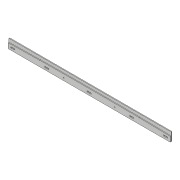
# Autodesk Inventor part: Guia eliptica
Saved by Autodesk Inventor 2019 (Build 230136000, 136)
## iProperties
Created: 2019-11-01
Part Number: Guia eliptica
Material: Generic
Document SubType Name: Modeling
Designer: Charlie
Density: 1 g/cm^3
Appearance: Default
Author: Charlie
Autodesk Inventor part; units mm, degrees
ref_plane "YZ Plane" through (0, 0, 0) normal (1, 0, 0) x (0, 1, 0)
ref_plane "XZ Plane" through (0, 0, 0) normal (0, 1, 0) x (-1, 0, 0)
ref_plane "XY Plane" through (0, 0, 0) normal (0, 0, 1) x (1, 0, 0)
sketch "Sketch1" plane through (0, 0, 0) normal (0, 0, 1) x (1, 0, 0)
  line L0 (-327.5, -120) -> (327.5, -120) construction
  line L1 (327.5, -120) -> (327.5, 120) construction
  line L2 (181.0324, 120) -> (-327.5, 120) construction
  line L3 (-327.5, 120) -> (-327.5, -120) construction
  line L4 (-327.5, -120) -> (327.5, 120) construction
  line L5 (327.5, -120) -> (-327.5, 120) construction
  line L6 (-327.5, 120) -> (-327.5, 122.5) construction
  line L7 (-145.4605, 120) -> (327.5, 120) construction
  line L8 (327.5, 120) -> (327.5, 125.5) construction
  line L9 (327.5, 125.5) -> (-327.5, 125.5) construction
  line L10 (-327.5, 125.5) -> (-327.5, 120) construction
  line L11 (-363.5951, 121.3114) -> (-639.7444, 121.118)
  line L12 (-327.5, 122.5) -> (-344.4955, 122.5)
  ellipse E0 centre (0, 122.5) end of major axis (-327.5, 122.5) minor radius 3 (327.5, 122.5) -> (-327.5, 122.5) ccw
  line L13 (-477.5, 120.5) -> (-292.2253, 123.8544)
  line L14 (-477.5, 120.5) -> (-477.5, 90.5)
  line L15 (-477.5, 90.5) -> (477.5, 90.5)
  line L16 (477.5, 90.5) -> (477.5, 120.5)
  line L17 (477.5, 120.5) -> (292.2253, 123.8544)
  point P0 (0, 0)
  dimension "d1" = 240
  dimension "d2" = 2.5
  dimension "d3" = 5.5
  dimension "d31" = 3
  dimension "d32" = 655
  dimension "d36" = 30
  dimension "d37" = 150
  dimension "d38" = 150
  dimension "d39" = 5
  constraints: 36 end point, 5 parallel, 4 horizontal, 4 perpendicular, 2 horizontal alignment, 2 midpoint, 2 point on line, 1 vertical, 8 other
  measures "d1" distance of L1.end L0.end
  measures "d2" distance of L6.end L2.end
  measures "d3" distance of L8.end L7.end
  measures "d31" distance from line of L6.end L9
  measures "d32" distance of L8.end L9.end
  measures "d36" distance of L13.start L14.end
  measures "d37" distance between parallel lines of L6 L14
  measures "d38" distance between parallel lines of L1 L16
  measures "d39" distance from line of L9 L16.end
extrude "Extrusion1" add sketch "Sketch1" along normal blind 5
sketch "Sketch9" plane through (0, 0, 0) normal (0, 0, -1) x (-1, 0, 0)
  line L0 (477.5, 120.5) -> (292.2253, 123.8544) projected
  ellipse E0 centre (0, 122.5) end of major axis (-327.5, 122.5) minor radius 3 (292.2253, 123.8544) -> (-292.2253, 123.8544) ccw projected
  line L1 (-292.2253, 123.8544) -> (-477.5, 120.5) projected
  line L2 (-477.5, 120.5) -> (-477.5, 90.5) projected
  line L3 (-477.5, 90.5) -> (477.5, 90.5) projected
  line L4 (477.5, 90.5) -> (477.5, 120.5) projected
  line L5 (477.5, 120.5) -> (477.5, 90.5) projected
  line L6 (477.5, 90.5) -> (-477.5, 90.5)
  line L7 (-477.5, 90.5) -> (-477.5, 140.5)
  line L8 (-477.5, 140.5) -> (477.5, 140.5)
  line L9 (477.5, 140.5) -> (477.5, 90.5)
  point P0 (0, 0)
  dimension "d40" = 50
  constraints: 8 end point, 2 parallel, 1 horizontal, 1 perpendicular, 1 other
  measures "d40" distance of L6.end L7.end
extrude "Extrusion7" add sketch "Sketch9" along normal blind 5 separate body
sketch "Sketch10" plane through (0, 0, 5) normal (0, 0, 1) x (1, 0, 0)
  line L0 (-10, 105.5) -> (10, 105.5) construction
  line L1 (-10, 102.5) -> (10, 102.5)
  line L2 (10, 108.5) -> (-10, 108.5)
  arc A0 (-10, 108.5) -> (-10, 102.5) centre (-10, 105.5) ccw
  arc A1 (10, 102.5) -> (10, 108.5) centre (10, 105.5) ccw
  line L3 (240, 105.5) -> (260, 105.5) construction
  line L4 (240, 102.5) -> (260, 102.5)
  line L5 (260, 108.5) -> (240, 108.5)
  arc A2 (240, 108.5) -> (240, 102.5) centre (240, 105.5) ccw
  arc A3 (260, 102.5) -> (260, 108.5) centre (260, 105.5) ccw
  line L6 (-260, 105.5) -> (-240, 105.5) construction
  line L7 (-260, 102.5) -> (-240, 102.5)
  line L8 (-240, 108.5) -> (-260, 108.5)
  arc A4 (-260, 108.5) -> (-260, 102.5) centre (-260, 105.5) ccw
  arc A5 (-240, 102.5) -> (-240, 108.5) centre (-240, 105.5) ccw
  line L9 (-477.5, 90.5) -> (477.5, 90.5) projected
  circle A6 centre (-150, 105.5) radius 2.75
  circle A7 centre (150, 105.5) radius 2.75
  line L10 (-460, 105.5) -> (-440, 105.5) construction
  line L11 (-460, 102.5) -> (-440, 102.5)
  line L12 (-440, 108.5) -> (-460, 108.5)
  arc A8 (-460, 108.5) -> (-460, 102.5) centre (-460, 105.5) ccw
  arc A9 (-440, 102.5) -> (-440, 108.5) centre (-440, 105.5) ccw
  line L13 (440, 105.5) -> (460, 105.5) construction
  line L14 (440, 102.5) -> (460, 102.5)
  line L15 (460, 108.5) -> (440, 108.5)
  arc A10 (440, 108.5) -> (440, 102.5) centre (440, 105.5) ccw
  arc A11 (460, 102.5) -> (460, 108.5) centre (460, 105.5) ccw
  point P0 (0, 0)
  point P1 (0, 105.5)
  point P2 (250, 105.5)
  point P3 (-250, 105.5)
  point P4 (-450, 105.5)
  point P5 (450, 105.5)
  dimension "d43" = 10
  dimension "d44" = 6
  dimension "d45" = 250
  dimension "d46" = 250
  dimension "d47" = 15
  dimension "d50" = 5.5
  dimension "d51" = 150
  dimension "d52" = 150
  dimension "d53" = 200
  dimension "d54" = 200
  constraints: 40 end point, 20 point on circle, 20 tangent, 12 centre point, 5 equal radius, 5 horizontal alignment, 5 midpoint, 5 parallel, 4 collinear, 4 point on line, 3 horizontal, 1 vertical alignment
  measures "d43" distance of point (0, 105.5) L0.end
  measures "d44" diameter of A1
  measures "d45" distance of point (250, 105.5) point (0, 105.5)
  measures "d46" distance of point (-250, 105.5) point (0, 105.5)
  measures "d47" distance between parallel lines of L9 L0
  measures "d50" diameter of A6
  measures "d51" distance of A6.centre point (0, 105.5)
  measures "d52" distance of A7.centre point (0, 105.5)
  measures "d53" distance of point (450, 105.5) point (250, 105.5)
  measures "d54" distance of point (-450, 105.5) point (-250, 105.5)
extrude "Extrusion8" cut sketch "Sketch10" against normal through all bodies 1 2
equation "\"d38\" = d37"
equation "\"d45\" = d46"
body "Solid8"
